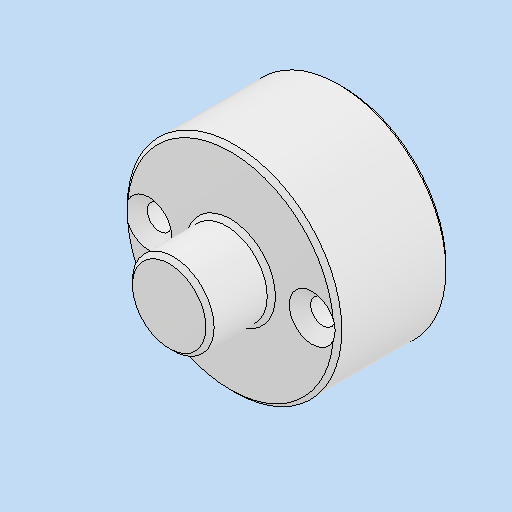
# Autodesk Inventor part: new-coupler
Saved by Autodesk Inventor 2025 (Build 290162000, 162)
## iProperties
Created: 2025-05-28
Part Number: new-coupler
Material: ABS Plastic
Document SubType Name: Modeling
Designer: kuzmin
Density: 1.06 g/cm^3
Appearance: Smooth - White
Author: kuzmin
Autodesk Inventor part; units mm, degrees
ref_plane "YZ Plane" through (0, 0, 0) normal (1, 0, 0) x (0, 1, 0)
ref_plane "XZ Plane" through (0, 0, 0) normal (0, 1, 0) x (-1, 0, 0)
ref_plane "XY Plane" through (0, 0, 0) normal (0, 0, 1) x (1, 0, 0)
sketch "Sketch1" plane through (0, 0, 0) normal (0, 0, 1) x (1, 0, 0)
  circle A0 centre (0, 0) radius 2.55
  circle A1 centre (0, 0) radius 10.5
  dimension "d0" = 21
  dimension "d1" = 5.1
  constraints: 2 centre point, 2 coincident
  measures "d0" diameter of A1
  measures "d1" diameter of A0
extrude "Extrusion1" add sketch "Sketch1" along normal blind 11
sketch "Sketch3" plane through (0, 0, 0) normal (0, 0, -1) x (-1, 0, 0)
  circle A0 centre (0, 0) radius 4.5
  dimension "d12" = 9
  constraints: 1 centre point, 1 coincident
  measures "d12" diameter of A0
extrude "Extrusion2" cut sketch "Sketch3" against normal blind 3
chamfer "Chamfer1" distance 1.93 angle 45 1 edges at (-2.55, 0, 3)
sketch "Sketch2" plane through (0, 0, 11) normal (0, 0, 1) x (1, 0, 0)
  circle A0 centre (0, 0) radius 8 construction
  point P0 (-8, 0)
  point P1 (8, 0)
  dimension "d4" = 16
  constraints: 2 horizontal alignment, 2 point on circle, 1 centre point, 1 coincident
  measures "d4" diameter of A0
hole "Hole1" at (-8, 0, 11) at (8, 0, 11) direction (0, 0, -1) diameter 2.4 end through all countersink diameter 4.5 countersink angle 90
sketch "Sketch6" plane through (0, 0, 11) normal (0, 0, 1) x (1, 0, 0)
  circle A0 centre (0, 0) radius 4
  dimension "d32" = 8
  constraints: 1 centre point, 1 coincident
  measures "d32" diameter of A0
extrude "Extrusion4" add sketch "Sketch6" along normal blind 6
chamfer "Chamfer3" distance 0.4 angle 45 4 edges at (-10.5, 0, 11) (-10.5, 0, 0) (-4, 0, 17) (4.5, 0, 0)
move faces "Move1" translate (0, 0, -6.1) faces at (0.6362, 0.5637, 11)
chamfer "Chamfer4" distance 0.4 angle 45 1 edges at (-4, 0, 11)
body "Solid1"
